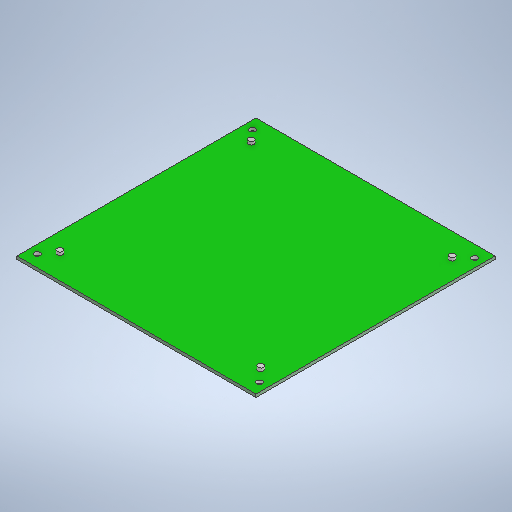
# Autodesk Inventor part: PCB
Saved by Autodesk Inventor 2025.2 (Build 292293000, 293)
## iProperties
Created: 2025-04-18
Part Number: PCB
Material: Generic
Document SubType Name: Modeling
Designer: 3lin2
Density: 1 g/cm^3
Appearance: Default
Author: 3lin2
Autodesk Inventor part; units mm, degrees
ref_plane "YZ Plane" through (0, 0, 0) normal (1, 0, 0) x (0, 1, 0)
ref_plane "XZ Plane" through (0, 0, 0) normal (0, 1, 0) x (-1, 0, 0)
ref_plane "XY Plane" through (0, 0, 0) normal (0, 0, 1) x (1, 0, 0)
sketch "Sketch1" plane through (0, 0, 0) normal (0, 1, 0) x (-1, 0, 0)
  line L0 (63.5, 63.5) -> (-63.5, 63.5)
  line L1 (-63.5, 63.5) -> (-63.5, -63.5)
  line L2 (-63.5, -63.5) -> (63.5, -63.5)
  line L3 (63.5, -63.5) -> (63.5, 63.5)
  point P0 (0, 0)
  dimension "d0" = 127
  dimension "d1" = 127
  dimension "d2" = 63.5
  dimension "d3" = 63.5
  constraints: 8 end point, 2 parallel, 1 horizontal, 1 perpendicular
  measures "d0" distance of L2.end L1.end
  measures "d1" distance of L1.end L0.end
  measures "d2" distance from line of L0 point (0, 0)
  measures "d3" distance from line of L3 point (0, 0)
extrude "Extrusion1" add sketch "Sketch1" along normal blind 1.5875
sketch "Sketch2" plane through (0, 1.5875, 0) normal (0, 1, 0) x (1, 0, 0)
  circle A0 centre (-59.055, 57.15) radius 1.524
  circle A1 centre (59.055, 57.15) radius 1.524
  circle A2 centre (59.055, -57.15) radius 1.524
  circle A3 centre (-59.055, -57.15) radius 1.524
  line L0 (63.5, 63.5) -> (-63.5, 63.5) projected
  line L1 (-63.5, 63.5) -> (-63.5, -63.5) projected
  point P0 (0, 0)
  dimension "d6" = 3.048
  dimension "d7" = 3.048
  dimension "d8" = 3.048
  dimension "d9" = 3.048
  dimension "d10" = 114.3
  dimension "d11" = 114.3
  dimension "d12" = 0
  dimension "d13" = 0
  dimension "d14" = 0
  dimension "d15" = 118.11
  dimension "d16" = 6.35
  dimension "d17" = 4.445
  constraints: 4 centre point
  measures "d6" diameter of A0
  measures "d7" diameter of A1
  measures "d8" diameter of A2
  measures "d9" diameter of A3
  measures "d10" distance of A3.centre A0.centre
  measures "d11" distance of A2.centre A1.centre
  measures "d12" horizontal distance of A2.centre A1.centre
  measures "d13" horizontal distance of A3.centre A0.centre
  measures "d14" vertical distance of A2.centre A3.centre
  measures "d15" distance of A1.centre A0.centre
  measures "d16" distance from line of A0.centre L0
  measures "d17" distance from line of L1 A3.centre
extrude "Extrusion2" cut sketch "Sketch2" against normal blind 1.5875
sketch "Sketch3" plane through (0, 1.5875, 0) normal (0, 1, 0) x (1, 0, 0)
  circle A0 centre (-53.34, 50.8) radius 1.524
  circle A1 centre (53.34, 50.8) radius 1.524
  circle A2 centre (53.34, -50.8) radius 1.524
  circle A3 centre (-53.34, -50.8) radius 1.524
  line L0 (63.5, 63.5) -> (-63.5, 63.5) projected
  line L1 (63.5, -63.5) -> (63.5, 63.5) projected
  point P0 (0, 0)
  dimension "d20" = 3.048
  dimension "d21" = 3.048
  dimension "d22" = 3.048
  dimension "d23" = 3.048
  dimension "d24" = 106.68
  dimension "d25" = 106.68
  dimension "d26" = 0
  dimension "d27" = 101.6
  dimension "d28" = 101.6
  dimension "d29" = 0
  dimension "d30" = 12.7
  dimension "d31" = 10.16
  constraints: 4 centre point
  measures "d20" diameter of A0
  measures "d21" diameter of A1
  measures "d22" diameter of A2
  measures "d23" diameter of A3
  measures "d24" distance of A1.centre A0.centre
  measures "d25" distance of A2.centre A3.centre
  measures "d26" vertical distance of A3.centre A2.centre
  measures "d27" distance of A3.centre A0.centre
  measures "d28" distance of A2.centre A1.centre
  measures "d29" horizontal distance of A3.centre A0.centre
  measures "d30" distance from line of L0 A0.centre
  measures "d31" distance from line of L1 A1.centre
extrude "Extrusion3" add sketch "Sketch3" along normal blind 1.5875
body "Solid1"
